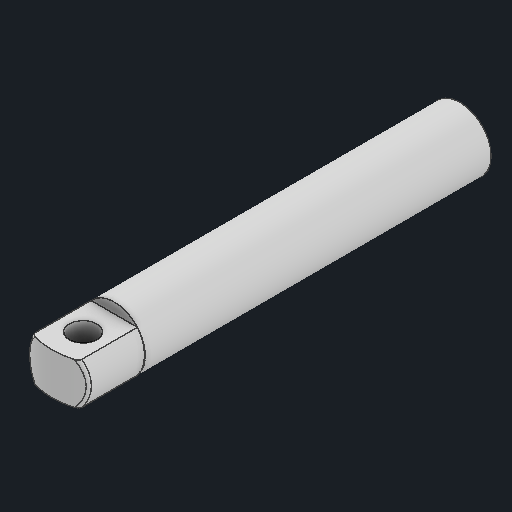
# Autodesk Inventor part: LA-T8-1215-50 105-64 Shaft
Saved by Autodesk Inventor 2025.2 (Build 292293000, 293)
## iProperties
Created: 2025-08-13
Part Number: LA-T8-1215-50 105-64 Shaft
Material: Generic
Document SubType Name: Modeling
Designer: valer
Density: 1 g/cm^3
Appearance: Default
Author: valer
Autodesk Inventor part; units mm, degrees
ref_plane "YZ Plane" through (0, 0, 0) normal (1, 0, 0) x (0, 1, 0)
ref_plane "XZ Plane" through (0, 0, 0) normal (0, 1, 0) x (-1, 0, 0)
ref_plane "XY Plane" through (0, 0, 0) normal (0, 0, 1) x (1, 0, 0)
sketch "Sketch1" plane through (0, 0, 0) normal (0, 0, 1) x (1, 0, 0)
  circle A0 centre (0, 0) radius 4.5
  dimension "d0" = 9
  constraints: 1 centre point, 1 coincident
  measures "d0" diameter of A0
extrude "Extrusion1" add sketch "Sketch1" along normal blind 50
sketch "Sketch2" plane through (0, 0, 50) normal (0, 0, 1) x (1, 0, 0)
  circle A0 centre (0, 0) radius 4.5 projected
  line L0 (-3.3541, 3) -> (3.3541, 3)
  line L1 (3.3541, 3) -> (3.3541, -3)
  line L2 (3.3541, -3) -> (-3.3541, -3)
  line L3 (-3.3541, -3) -> (-3.3541, 3)
  circle A1 centre (0, 0) radius 4.5 projected
  line L4 (-4.5, 0) -> (4.5, 0) construction
  arc A2 (-3.3541, 3) -> (-3.3541, -3) centre (0.5, 0) ccw
  line L5 (0, 3) -> (0, -3) construction
  arc A3 (3.3541, -3) -> (3.3541, 3) centre (-0.5, 0) ccw
  point P0 (-3.3541, 0)
  dimension "d3" = 6
  dimension "d4" = 0.5
  constraints: 12 end point, 9 point on circle, 3 midpoint, 2 centre point, 2 horizontal, 2 parallel, 1 perpendicular, 1 point on line, 1 symmetric about line, 1 other
  measures "d3" distance of L2.end L0.start
  measures "d4" distance of A0.centre A2.centre
extrude "Extrusion2" add sketch "Sketch2" along normal blind 9 contours L1 L2 L3 L0 | A3 L1 | L3 A2
sketch "Sketch3" plane through (-3.3541, -3, 50) normal (0, -1, 0) x (1, 0, 0)
  line L0 (7.7382, 0) -> (7.7382, 9) projected
  line L1 (-1.03, 0) -> (-1.03, 9) projected
  arc A0 (7.7382, 8) -> (-1.03, 8) centre (3.3541, -1.11) ccw
  line L2 (0, 9) -> (6.7082, 9) projected
  line L3 (0, 9) -> (-1.03, 9) projected
  line L4 (7.7382, 9) -> (6.7082, 9) projected
  point P0 (3.3541, -50)
  point P1 (3.3541, 9)
  dimension "d7" = 1
  dimension "d8" = 1
  constraints: 2 point on circle, 2 point on line, 1 centre point, 1 tangent
  measures "d7" distance of L1.end A0.end
  measures "d8" distance of L0.end A0.start
extrude "Extrusion3" cut sketch "Sketch3" against normal through all
fillet "Fillet1" radius 0.5 4 edges at (-4.1284, -1.5596, 58.1187) (-4.1284, 1.5596, 58.1187) (4.1284, 1.5596, 58.1187) (4.1284, -1.5596, 58.1187)
sketch "Sketch4" plane through (-3.3541, -3, 50) normal (0, -1, 0) x (1, 0, 0)
  line L0 (6.7082, 0) -> (0, 0) construction
  line L1 (3.3541, 0) -> (3.3541, 9) construction
  arc A0 (6.1913, 8.5937) -> (0.5169, 8.5937) centre (3.3541, -1.11) ccw construction
  circle A1 centre (3.3541, 4.5) radius 2
  line L2 (0, 0) -> (0, 8.0329) projected
  line L3 (0, 6.5) -> (6.7082, 6.5) construction
  line L4 (6.7082, 0) -> (6.7082, 8.0329) projected
  point P0 (3.3541, -50)
  point P1 (3.3541, 9)
  dimension "d12" = 4
  dimension "d13" = 2.5
  constraints: 4 end point, 2 midpoint, 2 point on circle, 2 point on line, 1 centre point, 1 horizontal, 1 tangent, 1 vertical
  measures "d12" diameter of A1
  measures "d13" distance from line of point (3.354, 9) L3
extrude "Extrusion4" cut sketch "Sketch4" against normal through all
body "Solid1"
